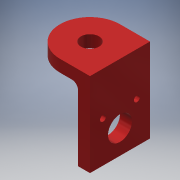
# Autodesk Inventor part: Corner Hinge
Saved by Autodesk Inventor 2017 (Build 210142000, 142)
## iProperties
Created: 2017-01-12
Part Number: Corner Hinge
Material: Generic
Document SubType Name: Modeling
Designer: Ben
Density: 1 g/cm^3
Appearance: Light Red
Author: Ben
Autodesk Inventor part; units mm, degrees
ref_plane "YZ Plane" through (0, 0, 0) normal (1, 0, 0) x (0, 1, 0)
ref_plane "XZ Plane" through (0, 0, 0) normal (0, 1, 0) x (-1, 0, 0)
ref_plane "XY Plane" through (0, 0, 0) normal (0, 0, 1) x (1, 0, 0)
sketch "Sketch1" plane through (0, 0, 0) normal (0, 0, 1) x (1, 0, 0)
  line L0 (0, 0) -> (0, 34.925)
  line L1 (-3.175, 38.1) -> (-25.4, 38.1)
  line L2 (-25.4, 38.1) -> (-25.4, 44.45)
  line L3 (-25.4, 44.45) -> (6.35, 44.45)
  line L4 (6.35, 44.45) -> (6.35, 0)
  line L5 (6.35, 0) -> (0, 0)
  arc A0 (0, 34.925) -> (-3.175, 38.1) centre (-3.175, 34.925) ccw
  point P0 (0, 38.1)
  dimension "d0" = 6.35
  dimension "d1" = 38.1
  dimension "d2" = 25.4
  dimension "d3" = 3.175
  constraints: 12 end point, 6 perpendicular, 2 point on circle, 2 point on line, 2 tangent, 1 centre point, 1 vertical
  measures "d0" distance of L4.end L0.start
  measures "d1" distance of L0.start point (0, 38.1)
  measures "d2" distance of point (0, 38.1) L1.end
  measures "d3" radius of A0
extrude "Extrusion1" add sketch "Sketch1" along normal blind 31.75
sketch "Sketch2" plane through (6.35, 0, 0) normal (1, 0, 0) x (0, 0, -1)
  line L0 (0, 38.1) -> (-31.75, 38.1) construction
  line L1 (0, 0) -> (-31.75, 0) construction
  line L2 (-15.875, 38.1) -> (-15.875, 0) construction
  line L3 (0, 0) -> (-31.75, 0) construction
  circle A0 centre (-15.875, 12.7) radius 6.35
  line L4 (0, 44.45) -> (-31.75, 44.45) construction
  line L5 (-15.875, 12.7) -> (-31.75, 28.575) construction
  line L6 (-31.75, 0) -> (-31.75, 44.45) construction
  circle A1 centre (-24.8553, 21.6803) radius 1.5875
  circle A2 centre (-6.8947, 21.6803) radius 1.5875
  dimension "d15" = 12.7
  dimension "d21" = 31.75
  dimension "d25" = 45
  dimension "d26" = 3.175
  dimension "d27" = 12.7
  constraints: 4 end point, 3 centre point, 3 point on line, 2 midpoint, 1 symmetric about line, 1 other
  measures "d15" diameter of A0
  measures "d21" distance from line of L5.start L4
  measures "d25" angle of L2 L5
  measures "d26" diameter of A1
  measures "d27" distance of L5.start A1.centre
extrude "Extrusion2" cut sketch "Sketch2" against normal through all
sketch "Sketch3" plane through (-25.4, 44.45, 0) normal (0, 1, 0) x (1, 0, 0)
  line L0 (0, 0) -> (0, -31.75) construction
  line L1 (0, 0) -> (0, -31.75) construction
  line L2 (0, -15.875) -> (15.875, -15.875) construction
  circle A0 centre (15.875, -15.875) radius 4.7625
  dimension "d17" = 9.525
  dimension "d18" = 15.875
  constraints: 2 end point, 1 centre point, 1 coincident, 1 horizontal, 1 midpoint
  measures "d17" diameter of A0
  measures "d18" distance of L2.start L2.end
extrude "Extrusion3" cut sketch "Sketch3" against normal through all
fillet "Fillet1" radius 15.875 2 edges at (-25.4, 41.275, 31.75) (-25.4, 41.275, 0)
equation "\"d7\" = d6"
equation "\"d6\" = 9.525"
body "Solid1"
